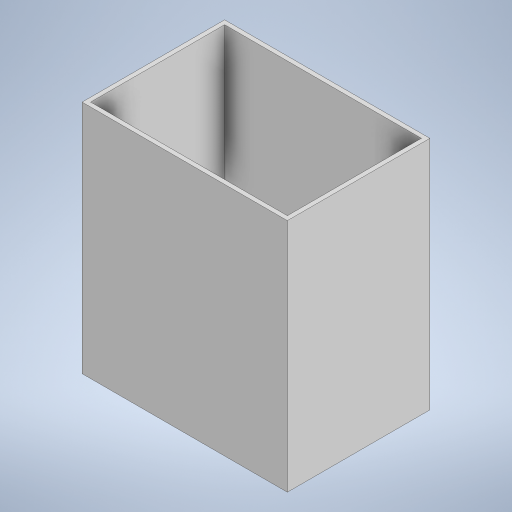
# Autodesk Inventor part: Caja1_SinOrificios
Saved by Autodesk Inventor 2024 (Build 280153000, 153)
## iProperties
Created: 2023-07-29
Part Number: Caja1_SinOrificios
Material: Genérico
Document SubType Name: Modeling
Designer: Det-Pc
Density: 1 g/cm^3
Appearance: Valor por defecto
Author: Det-Pc
Autodesk Inventor part; units mm, degrees
ref_plane "YZ Plane" through (0, 0, 0) normal (1, 0, 0) x (0, 1, 0)
ref_plane "XZ Plane" through (0, 0, 0) normal (0, 1, 0) x (-1, 0, 0)
ref_plane "XY Plane" through (0, 0, 0) normal (0, 0, 1) x (1, 0, 0)
sketch "Boceto3" plane through (0, 0, 0) normal (0, 1, 0) x (-1, 0, 0)
  line L0 (36, -25) -> (-36, -25)
  line L1 (-36, -25) -> (-36, 25)
  line L2 (-36, 25) -> (36, 25)
  line L3 (36, 25) -> (36, -25)
  point P0 (0, 0)
  point P1 (36, 0)
  point P2 (0, -25)
  dimension "d8" = 72
  dimension "d9" = 50
  constraints: 8 end point, 2 midpoint, 2 parallel, 1 horizontal, 1 horizontal alignment, 1 perpendicular, 1 vertical alignment
  measures "d8" distance of L1.end L2.end
  measures "d9" distance of L0.end L1.end
extrude "Extrusión2" add sketch "Boceto3" along normal blind 82.5
sketch "Boceto5" plane through (0, 82.5, 0) normal (0, 1, 0) x (1, 0, 0)
  line L0 (-34.5, -23.5) -> (34.5, -23.5)
  line L1 (34.5, -23.5) -> (34.5, 23.5)
  line L2 (34.5, 23.5) -> (-34.5, 23.5)
  line L3 (-34.5, 23.5) -> (-34.5, -23.5)
  line L4 (-36, 25) -> (-36, -25) projected
  line L5 (36, 25) -> (-36, 25) projected
  line L6 (36, -25) -> (36, 25) projected
  line L7 (-36, -25) -> (36, -25) projected
  point P0 (0, 0)
  dimension "d12" = 1.5
  dimension "d13" = 1.5
  dimension "d14" = 1.5
  dimension "d15" = 1.5
  constraints: 8 end point, 2 parallel, 1 horizontal, 1 perpendicular
  measures "d12" distance between parallel lines of L4 L3
  measures "d13" distance between parallel lines of L5 L2
  measures "d14" distance between parallel lines of L6 L1
  measures "d15" distance between parallel lines of L0 L7
extrude "Extrusión3" cut sketch "Boceto5" against normal blind 81 contours L3 L2 L1 L0
